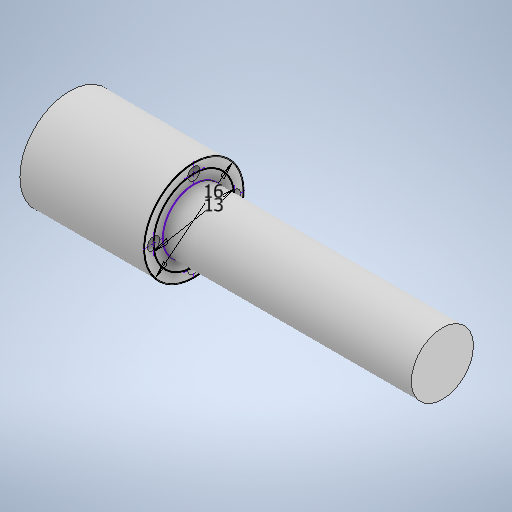
# Autodesk Inventor part: suspension2chassiscylindricalshaft
Saved by Autodesk Inventor 2025.4 (Build 294407000, 407)
## iProperties
Created: 2026-04-23
Part Number: suspension2chassiscylindricalshaft
Material: Generic
Document SubType Name: Modeling
Designer: hp
Density: 1 g/cm^3
Appearance: Default
Author: hp
Autodesk Inventor part; units mm, degrees
ref_plane "YZ Plane" through (0, 0, 0) normal (1, 0, 0) x (0, 1, 0)
ref_plane "XZ Plane" through (0, 0, 0) normal (0, 1, 0) x (-1, 0, 0)
ref_plane "XY Plane" through (0, 0, 0) normal (0, 0, 1) x (1, 0, 0)
sketch "Sketch1" plane through (0, 0, 0) normal (1, 0, 0) x (0, 1, 0)
  circle A0 centre (0, 0) radius 8
  circle A1 centre (0, 0) radius 5
  circle A2 centre (0, 0) radius 6.5
  point P0 (6.5, 0)
  point P1 (0, 6.5)
  point P2 (-6.5, 0)
  point P3 (0, -6.5)
  dimension "d0" = 16
  dimension "d5" = 13
  constraints: 4 point on circle, 3 centre point, 3 coincident
  measures "d0" diameter of A0
  measures "d5" diameter of A2
extrude "Extrusion1" add sketch "Sketch1" against normal blind 20 contours A0 | A1 | A2
extrude "Extrusion2" add sketch "Sketch1" along normal blind 40 contours A1
hole "Hole1" at (0, 6.5, 0) at (0, 0, 6.5) at (0, -6.5, 0) at (0, 0, -6.5) direction (-1, 0, 0) diameter 2 end through all
body "Solid1"
